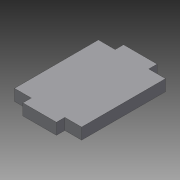
# Autodesk Inventor part: Frame_Lower_Vertical_Plate_C
Saved by Autodesk Inventor 2014 (Build 180170000, 170)
## iProperties
Created: 2014-08-27
Part Number: Frame_Lower_Vertical_Plate_C
Material: Generic
Document SubType Name: Modeling
Designer: ThatOtherGuy
Density: 1 g/cm^3
Appearance: Default
Author: ThatOtherGuy
Autodesk Inventor part; units mm, degrees
ref_plane "YZ Plane" through (0, 0, 0) normal (1, 0, 0) x (0, 1, 0)
ref_plane "XZ Plane" through (0, 0, 0) normal (0, 1, 0) x (-1, 0, 0)
ref_plane "XY Plane" through (0, 0, 0) normal (0, 0, 1) x (1, 0, 0)
sketch "Sketch1" plane through (0, 0, 0) normal (0, 0, 1) x (1, 0, 0)
  line L0 (0, 0) -> (10, 0)
  line L1 (10, 0) -> (10, -5)
  line L2 (10, -5) -> (30, -5)
  line L3 (30, -5) -> (30, 0)
  line L4 (30, 0) -> (40, 0)
  line L5 (40, 0) -> (40, 50)
  line L6 (40, 50) -> (30, 50)
  line L7 (30, 50) -> (30, 55)
  line L8 (30, 55) -> (10, 55)
  line L9 (10, 55) -> (10, 50)
  line L10 (10, 50) -> (0, 50)
  line L11 (0, 50) -> (0, 0)
  dimension "d0" = 20
  dimension "d1" = 10
  dimension "d2" = 5
  dimension "d3" = 50
  constraints: 24 end point, 8 parallel, 6 equal length, 2 collinear, 1 horizontal, 1 perpendicular
  measures "d0" distance of L7.end L8.end
  measures "d1" distance of L9.end L10.end
  measures "d2" distance of L8.end L9.end
  measures "d3" distance of L10.end L0.start
extrude "Extrusion1" add sketch "Sketch1" along normal blind 6.731
equation "\"d4\" = THICKB"
equation "\"THICKA\" = 3.175"
equation "\"THICKB\" = 6.731"
equation "\"THICKC\" = 12.7"
equation "\"MAGDIA\" = 9.5"
equation "\"BALLDIA\" = 12"
equation "\"THICKPLY\" = 5"
body "Solid1"
